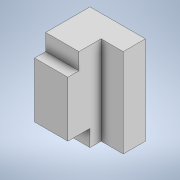
# Autodesk Inventor part: Martin-Probst-26673_obrazek_1
Saved by Autodesk Inventor 2021 (Build 250183000, 183)
## iProperties
Created: 2022-03-18
Part Number: Martin-Probst-26673_obrazek_1
Material: Všeobecné
Document SubType Name: Modeling
Designer: 26673
Density: 1 g/cm^3
Appearance: Výchozí
Author: 26673
Autodesk Inventor part; units mm, degrees
ref_plane "YZ Plane" through (0, 0, 0) normal (1, 0, 0) x (0, 1, 0)
ref_plane "XZ Plane" through (0, 0, 0) normal (0, 1, 0) x (-1, 0, 0)
ref_plane "XY Plane" through (0, 0, 0) normal (0, 0, 1) x (1, 0, 0)
sketch "Náčrt1" plane through (0, 0, 0) normal (1, 0, 0) x (0, 1, 0)
  line L0 (0, 0) -> (0, -50)
  line L1 (0, -50) -> (80, -50)
  line L2 (80, -50) -> (80, 0)
  line L3 (80, 0) -> (0, 0)
  dimension "d0" = 50
  dimension "d1" = 80
  dimension "d2" = 50
  constraints: 8 end point, 2 perpendicular, 1 vertical
  measures "d0" distance of L0.start L0.end
  measures "d1" distance of L0.end L1.end
  measures "d2" distance of L1.end L2.end
extrude "Vysunutí1" add sketch "Náčrt1" along normal blind 50
sketch "Náčrt2" plane through (50, 0, 0) normal (1, 0, 0) x (0, 0, -1)
  line L0 (0, 0) -> (20, 0)
  line L1 (0, 0) -> (50, 0) projected
  line L2 (20, 0) -> (20, 15)
  line L3 (20, 15) -> (0, 15)
  line L4 (0, 80) -> (0, 0) projected
  line L5 (0, 0) -> (0, 15)
  line L6 (0, 80) -> (10, 80)
  line L7 (50, 80) -> (0, 80) projected
  line L8 (10, 80) -> (10, 65)
  line L9 (10, 65) -> (0, 65)
  line L10 (0, 80) -> (0, 65)
  dimension "d5" = 20
  dimension "d6" = 15
  dimension "d7" = 10
  dimension "d8" = 15
  constraints: 16 end point, 4 point on line, 3 perpendicular, 2 vertical, 1 collinear
  measures "d5" distance of L0.start L0.end
  measures "d6" distance of L0.end L2.end
  measures "d7" distance of L4.start L6.end
  measures "d8" distance of L6.end L8.end
extrude "Vysunutí2" cut sketch "Náčrt2" against normal blind 50
sketch "Náčrt3" plane through (50, 0, 0) normal (1, 0, 0) x (0, 0, -1)
  line L0 (20, 0) -> (50, 0) projected
  line L1 (50, 0) -> (30, 0)
  line L2 (30, 0) -> (30, 80)
  line L3 (50, 80) -> (10, 80) projected
  line L4 (10, 80) -> (10, 65) projected
  line L5 (30, 80) -> (10, 80)
  line L6 (10, 80) -> (10, 65)
  line L7 (10, 65) -> (0, 65) projected
  line L8 (10, 65) -> (0, 65)
  line L9 (0, 15) -> (20, 15) projected
  line L10 (0, 65) -> (0, 15)
  line L11 (0, 15) -> (20, 15)
  line L12 (20, 15) -> (20, 0) projected
  line L13 (20, 15) -> (20, 0)
  line L14 (20, 0) -> (30, 0)
  point P0 (0, 0)
  dimension "d11" = 20
  constraints: 18 end point, 5 perpendicular, 1 collinear, 1 horizontal, 1 midpoint, 1 point on line
  measures "d11" distance of L0.end L1.end
extrude "Vysunutí3" cut sketch "Náčrt3" against normal blind 20
